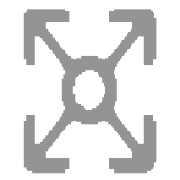
# Autodesk Inventor part: 2020Profile
Saved by Autodesk Inventor 2023 (Build 270158000, 158)
## iProperties
Created: 2023-08-13
Part Number: 2020Profile
Material: Aluminum 6061
Document SubType Name: Modeling
Designer: Felix
Standards Organization: DIN
Language: en-US
Size Designation: (Unnamed 1)
Categories: <MemberInstance><Categories><Category DisplayName="Structural Shapes" InternalName="089c4875-fa83-4c05-b084-43b9cc11f5ed" Mnemonic="GRDR"><CategoryParameter DisplayName="Mass per Length Unit" InternalName="0bb95a10-148f-4027-a459-38d7b056702a" Mnemonic="shpmass"/><CategoryParameter DisplayName="Section Area" InternalName="1ff91680-64b0-4202-b9a3-7fd3f94bba3b" Mnemonic="secarea"/><CategoryParameter DisplayName="Radius of Gyration (x)" InternalName="25778675-03e9-40c1-b6a8-4a9ed693320d" Mnemonic="gyrradx"/><CategoryParameter DisplayName="Torsional Rigidity Modulus" InternalName="26c1ec35-5026-4c63-ad0a-751cf684a536" Mnemonic="torrigmod"/><CategoryParameter DisplayName="Distance of the Center of Gravity X-X" InternalName="26c9bdb8-9c79-4b4f-a92e-8e197583c9c4" Mnemonic="grcendistX"/><CategoryParameter DisplayName="Legacy Member ID" InternalName="340afe4f-75d7-48d3-ab7d-943f3c3da468" Mnemonic="LegacyMemberID"/><CategoryParameter DisplayName="Base Length" InternalName="42e34263-8f20-4d0e-ad48-bf1385b87c24" Mnemonic="shplen"/><CategoryParameter DisplayName="Moment of Inertia (y)" InternalName="4b9f58ea-bced-460e-81ea-3d29ca5a49e3" Mnemonic="inermomy"/><CategoryParameter DisplayName="Moment of Inertia (x)" InternalName="4cd780bc-73d7-43ac-917a-579e5cbd684d" Mnemonic="inermomx"/><CategoryParameter DisplayName="Custom Base Point" InternalName="4f1d1b73-316d-484b-a3df-9cbabb16eb77" Mnemonic="shpBasePoint"/><CategoryParameter DisplayName="Shape Height" InternalName="50274e7d-5ac0-4796-92cb-c59e54983c67" Mnemonic="shpheig"/><CategoryParameter DisplayName="Section Module (y)" InternalName="59eaa5e9-d227-48dc-b6c1-6920f96e0f95" Mnemonic="secmody"/><CategoryParameter DisplayName="Section Designation" InternalName="5a64d034-428d-49c8-ba32-7619764de20f" Mnemonic="shpdes"/><CategoryParameter DisplayName="Section Module (x)" InternalName="72cfad18-cf51-4ed4-aaa7-c6b224f8419f" Mnemonic="secmodx"/><CategoryParameter DisplayName="Torsional Section Modulus" InternalName="7c55a8dc-8844-49f9-a867-cc677b30ec9a" Mnemonic="torsecmod"/><CategoryParameter DisplayName="Shape Width" InternalName="7c717d54-a18f-4666-b4d4-573cce22c62c" Mnemonic="shpwdth"/><CategoryParameter DisplayName="Second Shape Thickness" InternalName="9251a8e1-85fd-4e47-af99-afdb762317d9" Mnemonic="shpthick2"/><CategoryParameter DisplayName="FG Authored" InternalName="9c666724-f362-4ea7-ac62-f6a007de5c69" Mnemonic="shpFGAuto"/><CategoryParameter DisplayName="Distance of the Center of Gravity Y-Y" InternalName="bcc4fb17-7af4-436a-8f8c-d0aa3b0248c5" Mnemonic="grcendistY"/><CategoryParameter DisplayName="Radius of Gyration (y)" InternalName="bfa18ebe-1636-4dbe-8d42-b263e0b73184" Mnemonic="gyrrady"/><CategoryParameter DisplayName="Shape Thickness" InternalName="d109cf76-8eb4-42fc-9800-4409734adc67" Mnemonic="shpthick"/><CategoryParameter DisplayName="Coefficient of Shear Displacement" InternalName="de4c90c6-aaa8-468f-a335-6737b311b5d3" Mnemonic="shdispc"/><Category DisplayName="Other" InternalName="f02205ff-2390-476f-921c-0b3185f88e84" Mnemonic="OTHSHP"><CategoryParameter DisplayName="Moment of Inertia (y)" InternalName="044c654e-f649-48ac-84cc-650a29ae31ca" Mnemonic="inermomy"/><CategoryParameter DisplayName="Shape Thickness" InternalName="12b1a788-9233-48fd-a933-2df8ff42b15f" Mnemonic="shpthick"/><CategoryParameter DisplayName="Mass per Length Unit" InternalName="2fd289d6-9394-4d2d-97e6-6659d7d4551d" Mnemonic="shpmass"/><CategoryParameter DisplayName="Radius of Gyration (y)" InternalName="743e1dfe-1bba-408b-b985-cf752b207386" Mnemonic="gyrrady"/><CategoryParameter DisplayName="Section Module (y)" InternalName="88b8bff9-a616-4028-93d5-ed4f79680d13" Mnemonic="secmody"/><CategoryParameter DisplayName="Section Area" InternalName="c46ecdf8-b6eb-4db9-8b25-30258930c1e3" Mnemonic="secarea"/><CategoryParameter DisplayName="Section Module (x)" InternalName="cac70804-9d39-43bb-be17-56ea1f39a6c2" Mnemonic="secmodx"/><CategoryParameter DisplayName="Moment of Inertia (x)" InternalName="ec6737bc-264f-43ed-b0bd-f6d410c2718d" Mnemonic="inermomx"/><CategoryParameter DisplayName="Radius of Gyration (x)" InternalName="ee72c61e-565e-4fd6-b448-66e1e1abcb7e" Mnemonic="gyrradx"/></Category></Category><Category DisplayName="DataType" InternalName="23b78d0f-2648-40c6-8793-ca6db495c9e8" Mnemonic="DATATYPE"><CategoryParameter DisplayName="DisplayName" InternalName="05415f3d-3907-474b-a020-eb9d644f4cf3" Mnemonic="DISPLAYNAME"/><CategoryParameter DisplayName="Standard" InternalName="0c0a119c-1e12-4c84-803f-101930972f5e" Mnemonic="STANDARD"/><CategoryParameter DisplayName="Description" InternalName="13903e3d-64b1-4950-80da-f627842ea37f" Mnemonic="DESCRIPTION"/><CategoryParameter DisplayName="Designation" InternalName="2675968c-4ce5-49e0-a4f5-552d29089031" Mnemonic="DESIGNATION"/><CategoryParameter DisplayName="Default Row" InternalName="2af9ec52-faaa-4026-b378-f9fa4afca842" Mnemonic="DEFAULTROW"/><CategoryParameter DisplayName="Folder Name" InternalName="3f06958e-8713-4116-9be7-ed6184ecc97b" Mnemonic="FOLDERNAME"/><CategoryParameter DisplayName="Revision Guid" InternalName="45a75005-10b1-4dfc-8d6d-dfe629f0b93c" Mnemonic="REVISIONGUID"/><CategoryParameter DisplayName="FileName" InternalName="8b46a4cc-9585-4fed-90c3-899f57e09a73" Mnemonic="FILENAME"/><CategoryParameter DisplayName="StdsOrg" InternalName="8f5914e1-4693-403f-8ab5-d37768198c9d" Mnemonic="STDSORG"/><CategoryParameter DisplayName="Family Version" InternalName="914462f6-6e19-4b14-ba84-155b9680b1d0" Mnemonic="FAMILYREVISION"/><CategoryParameter DisplayName="Standard Revision" InternalName="91d5a463-65c2-4fde-b823-3b7fea5e8e17" Mnemonic="STANDARDREVISION"/><CategoryParameter DisplayName="Member Revision" InternalName="a65d44b9-392f-4f4f-857b-e4b3d54996fe" Mnemonic="MEMBERREVISION"/><CategoryParameter DisplayName="ClipFormat" InternalName="bc51e27b-3422-4e78-93ef-cec197ddf230" Mnemonic="CLIPFORMAT"/><CategoryParameter DisplayName="Manufacturer" InternalName="cd6c7a72-a28a-4e50-99a9-2c7f4e13e5ad" Mnemonic="MANUFACTURER"/><CategoryParameter DisplayName="InternalName" InternalName="cf1d0246-76d9-4b4a-8305-fa0409afb5c1" Mnemonic="INTERNALNAME"/><CategoryParameter DisplayName="IsMetric" InternalName="e2385c5b-1ea4-4823-96a8-8de651266ec3" Mnemonic="ISMETRIC"/><Category DisplayName="Part" InternalName="c0e0b642-3bcb-4cc8-9e80-f96d35c4afa4" Mnemonic="PART"><CategoryParameter DisplayName="Part Number" InternalName="016b6077-bfbe-49bd-92c9-d8d59c39c941" Mnemonic="PARTNUMBER"/><CategoryParameter DisplayName="Stock Number" InternalName="4dba7c1c-e26c-444e-836c-b08b433409a8" Mnemonic="STOCKNUMBER"/><CategoryParameter DisplayName="Material Key" InternalName="5c9a8adb-dd2b-4535-b97f-0a94a95fe41f" Mnemonic="MATERIALKEY"/><CategoryParameter DisplayName="Material" InternalName="818a152a-d3c3-49ca-80ee-df7d91421b8e" Mnemonic="MATERIAL"/></Category></Category></Categories><FamilyTemplate Id="2020Profile"><FamilyTemplateParameters><FamilyTemplateParameter ObjectType="kUserParameterObject" ValueType="xs:double" Id="12" ObjectReferenceKey="LENGTH"/><FamilyTemplateParameter ObjectType="kPartComponentDefinitionObject" ValueType="xs:string" Id="23" SubObjectId="Material"/><FamilyTemplateParameter ObjectType="kPropertyObject" ValueType="xs:string" Id="26" ObjectReferenceKey="{32853F0F-3444-11d1-9E93-0060B03C1CA6}" SubObjectId="5"/><FamilyTemplateParameter ObjectType="kPropertyObject" ValueType="xs:string" Id="27" ObjectReferenceKey="{32853F0F-3444-11d1-9E93-0060B03C1CA6}" SubObjectId="52"/></FamilyTemplateParameters></FamilyTemplate><CategoryParameterMap><ParamToTemplateMap><ParamToTemplate CategoryParameter="//CategoryParameter[@InternalName='cf1d0246-76d9-4b4a-8305-fa0409afb5c1']" ConstantValue="705beb49-5b22-4cca-9ddd-617f30b7a52f"/><ParamToTemplate CategoryParameter="//CategoryParameter[@InternalName='45a75005-10b1-4dfc-8d6d-dfe629f0b93c']" ConstantValue="0819a46a-e16f-457d-87dc-9bd2e8dff1b5"/><ParamToTemplate CategoryParameter="//CategoryParameter[@InternalName='3f06958e-8713-4116-9be7-ed6184ecc97b']" ConstantValue="2020"/><ParamToTemplate CategoryParameter="//CategoryParameter[@InternalName='8f5914e1-4693-403f-8ab5-d37768198c9d']" ConstantValue="DIN"/><ParamToTemplate CategoryParameter="//CategoryParameter[@InternalName='0c0a119c-1e12-4c84-803f-101930972f5e']" TemplateParameter="18"/><ParamToTemplate CategoryParameter="//CategoryParameter[@InternalName='91d5a463-65c2-4fde-b823-3b7fea5e8e17']" TemplateParameter="19"/><ParamToTemplate CategoryParameter="//CategoryParameter[@InternalName='cd6c7a72-a28a-4e50-99a9-2c7f4e13e5ad']" TemplateParameter="20"/><ParamToTemplate CategoryParameter="//CategoryParameter[@InternalName='13903e3d-64b1-4950-80da-f627842ea37f']" TemplateParameter="22"/><ParamToTemplate CategoryParameter="//CategoryParameter[@InternalName='05415f3d-3907-474b-a020-eb9d644f4cf3']" ConstantValue="2020"/><ParamToTemplate CategoryParameter="//CategoryParameter[@InternalName='914462f6-6e19-4b14-ba84-155b9680b1d0']" ConstantValue="11"/><ParamToTemplate CategoryParameter="//CategoryParameter[@InternalName='bc51e27b-3422-4e78-93ef-cec197ddf230']" ConstantValue="CF_INVENTOR.STDPARTS"/><ParamToTemplate CategoryParameter="//CategoryParameter[@InternalName='e2385c5b-1ea4-4823-96a8-8de651266ec3']" ConstantValue="true"/><ParamToTemplate CategoryParameter="//CategoryParameter[@InternalName='2af9ec52-faaa-4026-b378-f9fa4afca842']" ConstantValue="1"/><ParamToTemplate CategoryParameter="//CategoryParameter[@InternalName='9c666724-f362-4ea7-ac62-f6a007de5c69']" ConstantValue="1"/><ParamToTemplate CategoryParameter="//CategoryParameter[@InternalName='8b46a4cc-9585-4fed-90c3-899f57e09a73']" ConstantValue="100"/><ParamToTemplate CategoryParameter="//CategoryParameter[@InternalName='a65d44b9-392f-4f4f-857b-e4b3d54996fe']" ConstantValue="4603198c-81e0-4cc1-864e-f1b7f9832bd5"/><ParamToTemplate CategoryParameter="//CategoryParameter[@InternalName='a65d44b9-392f-4f4f-857b-e4b3d54996fe']" ConstantValue="4603198c-81e0-4cc1-864e-f1b7f9832bd5"/><ParamToTemplate CategoryParameter="//CategoryParameter[@InternalName='2675968c-4ce5-49e0-a4f5-552d29089031']" TemplateParameter="27"/><ParamToTemplate CategoryParameter="//CategoryParameter[@InternalName='42e34263-8f20-4d0e-ad48-bf1385b87c24']" TemplateParameter="12"/><ParamToTemplate CategoryParameter="//CategoryParameter[@InternalName='818a152a-d3c3-49ca-80ee-df7d91421b8e']" TemplateParameter="23"/><ParamToTemplate CategoryParameter="//CategoryParameter[@InternalName='016b6077-bfbe-49bd-92c9-d8d59c39c941']" TemplateParameter="26"/></ParamToTemplateMap></CategoryParameterMap></MemberInstance>
Density: 2.7 g/cm^3
Appearance: Aluminum - Flat
_CCFamilyDisplayName: 2020
_FrameMemberDoc: Frame Member File
_Version: 15.0.0
_GetPNFromCC: 1
IsCustomPart: 1
Author: Felix
G_L: 200,000 mm
G_W: 20,000 mm
G_H: 20,000 mm
Autodesk Inventor part; units mm, degrees
ref_plane "YZ Plane" through (0, 0, 0) normal (1, 0, 0) x (0, 1, 0)
ref_plane "Start Plane" through (0, 0, 0) normal (0, 0, 1) x (1, 0, 0)
ref_plane "End Plane" through (0, 0, 200) normal (0, 0, 1) x (1, 0, 0)
sketch "Sketch" plane through (0, 0, 0) normal (0, 0, 1) x (1, 0, 0)
  circle A0 centre (0, 0) radius 2.5
  circle A1 centre (0, 0) radius 4.2 construction
  line L0 (10, -10) -> (-10, -10) construction
  line L1 (-10, -10) -> (-10, 10) construction
  line L2 (-10, 10) -> (10, 10) construction
  line L3 (10, 10) -> (10, -10) construction
  line L4 (10, -10) -> (-10, 10) construction
  line L5 (-10, -10) -> (10, 10) construction
  line L6 (-4.1658, 3.1759) -> (-7.7464, 6.7565)
  line L7 (-10, 8.8) -> (-10, 3.95)
  line L8 (-10, 3.95) -> (-9.6, 3.95)
  line L9 (-9.6, 3.95) -> (-9.6, 3.2)
  line L10 (-9.6, 3.2) -> (-8.6, 3.2)
  line L11 (-8.6, 3.2) -> (-8.6, 6.4029)
  line L12 (-10, 0) -> (0, 0) construction
  line L13 (-8.8, 10) -> (-3.95, 10)
  line L14 (-3.95, 10) -> (-3.95, 9.6)
  line L15 (-3.95, 9.6) -> (-3.2, 9.6)
  line L16 (-3.2, 9.6) -> (-3.2, 8.6)
  line L17 (-3.2, 8.6) -> (-6.4029, 8.6)
  arc A2 (-8.8, 10) -> (-10, 8.8) centre (-8.8, 8.8) ccw
  arc A3 (-6.4029, 8.6) -> (-6.7565, 7.7464) centre (-6.4029, 8.1) ccw
  arc A4 (-7.7464, 6.7565) -> (-8.6, 6.4029) centre (-8.1, 6.4029) ccw
  arc A5 (-3.8668, 1.6394) -> (-4.2, 0) centre (0, 0) ccw
  arc A6 (-3.8668, 1.6394) -> (-4.1658, 3.1759) centre (-5.1558, 2.1859) ccw
  line L18 (-3.1759, 4.1658) -> (-6.7565, 7.7464)
  arc A7 (0, 4.2) -> (-1.6394, 3.8668) centre (0, 0) ccw
  arc A8 (-3.1759, 4.1658) -> (-1.6394, 3.8668) centre (-2.1859, 5.1558) ccw
  line L19 (-3.2, -9.6) -> (-3.2, -8.6)
  line L20 (-3.2, -8.6) -> (-6.4029, -8.6)
  line L21 (-8.8, -10) -> (-3.95, -10)
  arc A9 (-1.6394, -3.8668) -> (-3.1759, -4.1658) centre (-2.1859, -5.1558) ccw
  line L22 (-3.1759, -4.1658) -> (-6.7565, -7.7464)
  line L23 (0, -10) -> (0, 0) construction
  arc A10 (-4.1658, -3.1759) -> (-3.8668, -1.6394) centre (-5.1558, -2.1859) ccw
  line L24 (-4.1658, -3.1759) -> (-7.7464, -6.7565)
  line L25 (-3.95, -9.6) -> (-3.2, -9.6)
  line L26 (-3.95, -10) -> (-3.95, -9.6)
  arc A11 (-1.6394, -3.8668) -> (0, -4.2) centre (0, 0) ccw
  arc A12 (-4.2, 0) -> (-3.8668, -1.6394) centre (0, 0) ccw
  line L27 (-9.6, -3.95) -> (-9.6, -3.2)
  arc A13 (-6.7565, -7.7464) -> (-6.4029, -8.6) centre (-6.4029, -8.1) ccw
  arc A14 (-8.6, -6.4029) -> (-7.7464, -6.7565) centre (-8.1, -6.4029) ccw
  line L28 (-8.6, -3.2) -> (-8.6, -6.4029)
  line L29 (-9.6, -3.2) -> (-8.6, -3.2)
  line L30 (-10, -3.95) -> (-9.6, -3.95)
  line L31 (-10, -8.8) -> (-10, -3.95)
  arc A15 (-10, -8.8) -> (-8.8, -10) centre (-8.8, -8.8) ccw
  line L32 (9.6, -3.2) -> (8.6, -3.2)
  line L33 (8.6, -3.2) -> (8.6, -6.4029)
  line L34 (10, -8.8) -> (10, -3.95)
  arc A16 (3.8668, -1.6394) -> (4.1658, -3.1759) centre (5.1558, -2.1859) ccw
  line L35 (4.1658, -3.1759) -> (7.7464, -6.7565)
  line L36 (10, 0) -> (0, 0) construction
  arc A17 (3.1759, -4.1658) -> (1.6394, -3.8668) centre (2.1859, -5.1558) ccw
  line L37 (3.1759, -4.1658) -> (6.7565, -7.7464)
  line L38 (9.6, -3.95) -> (9.6, -3.2)
  line L39 (10, -3.95) -> (9.6, -3.95)
  arc A18 (3.8668, -1.6394) -> (4.2, 0) centre (0, 0) ccw
  arc A19 (0, -4.2) -> (1.6394, -3.8668) centre (0, 0) ccw
  line L40 (3.95, -9.6) -> (3.2, -9.6)
  arc A20 (7.7464, -6.7565) -> (8.6, -6.4029) centre (8.1, -6.4029) ccw
  arc A21 (6.4029, -8.6) -> (6.7565, -7.7464) centre (6.4029, -8.1) ccw
  line L41 (3.2, -8.6) -> (6.4029, -8.6)
  line L42 (3.2, -9.6) -> (3.2, -8.6)
  line L43 (3.95, -10) -> (3.95, -9.6)
  line L44 (8.8, -10) -> (3.95, -10)
  arc A22 (8.8, -10) -> (10, -8.8) centre (8.8, -8.8) ccw
  line L45 (3.2, 9.6) -> (3.2, 8.6)
  line L46 (3.2, 8.6) -> (6.4029, 8.6)
  line L47 (8.8, 10) -> (3.95, 10)
  arc A23 (1.6394, 3.8668) -> (3.1759, 4.1658) centre (2.1859, 5.1558) ccw
  line L48 (3.1759, 4.1658) -> (6.7565, 7.7464)
  line L49 (0, 10) -> (0, 0) construction
  arc A24 (4.1658, 3.1759) -> (3.8668, 1.6394) centre (5.1558, 2.1859) ccw
  line L50 (4.1658, 3.1759) -> (7.7464, 6.7565)
  line L51 (3.95, 9.6) -> (3.2, 9.6)
  line L52 (3.95, 10) -> (3.95, 9.6)
  arc A25 (1.6394, 3.8668) -> (0, 4.2) centre (0, 0) ccw
  arc A26 (4.2, 0) -> (3.8668, 1.6394) centre (0, 0) ccw
  line L53 (9.6, 3.95) -> (9.6, 3.2)
  arc A27 (6.7565, 7.7464) -> (6.4029, 8.6) centre (6.4029, 8.1) ccw
  arc A28 (8.6, 6.4029) -> (7.7464, 6.7565) centre (8.1, 6.4029) ccw
  line L54 (8.6, 3.2) -> (8.6, 6.4029)
  line L55 (9.6, 3.2) -> (8.6, 3.2)
  line L56 (10, 3.95) -> (9.6, 3.95)
  line L57 (10, 8.8) -> (10, 3.95)
  arc A29 (10, 8.8) -> (8.8, 10) centre (8.8, 8.8) ccw
  point P0 (-3.4233, 2.4333)
  point P1 (-8.6, 7.6101)
  point P2 (-7.6101, 8.6)
  point P3 (-7.6101, -8.6)
  point P4 (-10, -10)
  point P5 (-2.4333, -3.4233)
  point P6 (-8.6, -7.6101)
  point P7 (8.6, -7.6101)
  point P8 (10, -10)
  point P9 (3.4233, -2.4333)
  point P10 (7.6101, -8.6)
  point P11 (7.6101, 8.6)
  point P12 (10, 10)
  point P13 (2.4333, 3.4233)
  point P14 (8.6, 7.6101)
  point P15 (-4.2, 0)
  point P16 (0, -4.2)
  point P17 (4.2, 0)
  point P18 (0, 4.2)
  dimension "d8" = 5
  dimension "d9" = 8.4
  dimension "d10" = 20
  dimension "d11" = 20
  dimension "d13" = 1.4
  dimension "d14" = 3.2
  dimension "d15" = 3.95
  dimension "d16" = 0.4
  dimension "d18" = 1.2
  dimension "d19" = 0.5
  dimension "d20" = 1.4
  dimension "d21" = 1.4
  dimension "d24" = 360
  constraints: 116 end point, 59 point on circle, 30 centre point, 29 point on line, 10 coincident, 9 symmetric about line, 8 tangent, 4 perpendicular, 3 horizontal, 3 midpoint, 3 parallel, 2 equal radius, 218 other
  measures "d8" diameter of A0
  measures "d9" diameter of A1
  measures "d10" distance of L1.end L2.end
  measures "d11" distance of L0.end L1.end
  measures "d13" distance between parallel lines of L7 L11
  measures "d14" distance between parallel lines of L12 L10
  measures "d15" distance between parallel lines of L12 L8
  measures "d16" distance between parallel lines of L9 L1
  measures "d18" radius of A2
  measures "d19" radius of A3
  measures "d20" radius of A6
  measures "d21" distance between parallel lines of L18 L6
extrude "Body" add sketch "Sketch" along normal up to surface (200 mm away) from surface at 0
sketch "Sketch11" plane through (0, 0, 0) normal (0, 0, 1) x (1, 0, 0)
  line L0 (0, 0) -> (10, 0)
ref_plane "Work Plane11" through (0, 0, 0) normal (0, -1, 0) x (1, 0, 0)
sketch "Sketch12" plane through (0, 0, 0) normal (0, -1, 0) x (1, 0, 0)
  line L0 (-2, 0) -> (12, 0)
  line L1 (-2, 200) -> (12, 200)
  dimension "d53" = 200
  measures "d53" distance between parallel lines of L0 L1
equation "\"G_OFFSET_START\" = 0"
equation "\"G_OFFSET_END\" = 0"
equation "\"G_L\" = d53"
equation "\"G_OFFSET_START1\" = 0"
equation "\"G_OFFSET_END1\" = 0"
equation "\"G_OFFSET_START2\" = 0"
equation "\"G_OFFSET_END2\" = 0"
body "Solid3"
